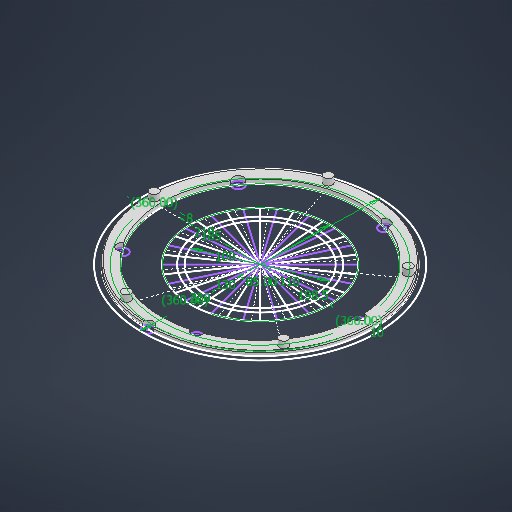
# Autodesk Inventor part: Aparatus_Motion_Conveyer
Saved by Autodesk Inventor 2026.2 (Build 302298000, 298)
## iProperties
Created: 2025-12-30
Part Number: Aparatus_Motion_Conveyer
Material: Generic
Document SubType Name: Modeling
Designer: Cobble
Density: 1 g/cm^3
Appearance: Default
Author: Cobble
Autodesk Inventor part; units mm, degrees
ref_plane "YZ Plane" through (0, 0, 0) normal (1, 0, 0) x (0, 1, 0)
ref_plane "XZ Plane" through (0, 0, 0) normal (0, 1, 0) x (-1, 0, 0)
ref_plane "XY Plane" through (0, 0, 0) normal (0, 0, 1) x (1, 0, 0)
sketch "Sketch1" plane through (0, 0, 0) normal (0, 0, 1) x (1, 0, 0)
  circle A0 centre (0, 0) radius 99.25
  circle A1 centre (-99.25, 0) radius 4
  circle A2 centre (0, 0) radius 92.5
  circle A3 centre (0, 0) radius 105
  line L0 (0, 0) -> (-99.25, 0) construction
  line L1 (0, 0) -> (-30.6699, -94.3924) construction
  circle A4 centre (-30.6699, -94.3924) radius 4
  line L2 (0, 0) -> (80.2949, -58.3377) construction
  circle A5 centre (80.2949, -58.3377) radius 4
  line L3 (0, 0) -> (80.2949, 58.3377) construction
  circle A6 centre (80.2949, 58.3377) radius 4
  line L4 (0, 0) -> (-30.6699, 94.3924) construction
  circle A7 centre (-30.6699, 94.3924) radius 4
  circle A8 centre (0, 0) radius 50
  circle A9 centre (0, 0) radius 55
  circle A10 centre (0, 0) radius 65
  line L5 (0, 0) -> (0, -65) construction
  line L6 (0, 0) -> (5.6651, -64.7527)
  line L7 (0, 0) -> (65, 0) construction
  line L8 (0, 0) -> (-5.6651, -64.7527)
  line L9 (0, 0) -> (16.8232, -62.7852)
  line L10 (0, 0) -> (22.2313, -61.08) construction
  line L11 (0, 0) -> (27.4702, -58.91)
  line L12 (0, 0) -> (37.2825, -53.2449)
  line L13 (0, 0) -> (41.7812, -49.7929) construction
  line L14 (0, 0) -> (45.9619, -45.9619)
  line L15 (0, 0) -> (53.2449, -37.2825)
  line L16 (0, 0) -> (56.2917, -32.5) construction
  line L17 (0, 0) -> (58.91, -27.4702)
  line L18 (0, 0) -> (62.7852, -16.8232)
  line L19 (0, 0) -> (64.0125, -11.2871) construction
  line L20 (0, 0) -> (64.7527, -5.6651)
  line L21 (0, 0) -> (64.7527, 5.6651)
  line L22 (0, 0) -> (64.0125, 11.2871) construction
  line L23 (0, 0) -> (62.7852, 16.8232)
  line L24 (0, 0) -> (58.91, 27.4702)
  line L25 (0, 0) -> (56.2917, 32.5) construction
  line L26 (0, 0) -> (53.2449, 37.2825)
  line L27 (0, 0) -> (45.9619, 45.9619)
  line L28 (0, 0) -> (41.7812, 49.7929) construction
  line L29 (0, 0) -> (37.2825, 53.2449)
  line L30 (0, 0) -> (27.4702, 58.91)
  line L31 (0, 0) -> (22.2313, 61.08) construction
  line L32 (0, 0) -> (16.8232, 62.7852)
  line L33 (0, 0) -> (5.6651, 64.7527)
  line L34 (0, 0) -> (0, 65) construction
  line L35 (0, 0) -> (-5.6651, 64.7527)
  line L36 (0, 0) -> (-16.8232, 62.7852)
  line L37 (0, 0) -> (-22.2313, 61.08) construction
  line L38 (0, 0) -> (-27.4702, 58.91)
  line L39 (0, 0) -> (-37.2825, 53.2449)
  line L40 (0, 0) -> (-41.7812, 49.7929) construction
  line L41 (0, 0) -> (-45.9619, 45.9619)
  line L42 (0, 0) -> (-53.2449, 37.2825)
  line L43 (0, 0) -> (-56.2917, 32.5) construction
  line L44 (0, 0) -> (-58.91, 27.4702)
  line L45 (0, 0) -> (-62.7852, 16.8232)
  line L46 (0, 0) -> (-64.0125, 11.2871) construction
  line L47 (0, 0) -> (-64.7527, 5.6651)
  line L48 (0, 0) -> (-64.7527, -5.6651)
  line L49 (0, 0) -> (-64.0125, -11.2871) construction
  line L50 (0, 0) -> (-62.7852, -16.8232)
  line L51 (0, 0) -> (-58.91, -27.4702)
  line L52 (0, 0) -> (-56.2917, -32.5) construction
  line L53 (0, 0) -> (-53.2449, -37.2825)
  line L54 (0, 0) -> (-45.9619, -45.9619)
  line L55 (0, 0) -> (-41.7812, -49.7929) construction
  line L56 (0, 0) -> (-37.2825, -53.2449)
  line L57 (0, 0) -> (-27.4702, -58.91)
  line L58 (0, 0) -> (-22.2313, -61.08) construction
  line L59 (0, 0) -> (-16.8232, -62.7852)
  circle A11 centre (0, 0) radius 110
  circle A12 centre (0, -105) radius 5
  circle A13 centre (92.5, 0) radius 5
  circle A14 centre (28.5841, 87.9727) radius 5
  circle A15 centre (-74.8341, 54.3701) radius 5
  circle A16 centre (-74.8341, -54.3701) radius 5
  circle A17 centre (28.5841, -87.9727) radius 5
  point P0 (0, -50)
  point P1 (53.1259, -14.235)
  point P2 (49.8469, -23.244)
  point P3 (45.0534, -31.5467)
  point P4 (38.8909, -38.8909)
  point P5 (31.5467, -45.0534)
  point P6 (23.244, -49.8469)
  point P7 (14.235, -53.1259)
  point P8 (4.7936, -54.7907)
  point P9 (-14.235, -53.1259)
  point P10 (-4.7936, -54.7907)
  point P11 (-23.244, -49.8469)
  point P12 (-31.5467, -45.0534)
  point P13 (-38.8909, -38.8909)
  point P14 (-45.0534, -31.5467)
  point P15 (-49.8469, -23.244)
  point P16 (-53.1259, -14.235)
  point P17 (-54.7907, -4.7936)
  point P18 (-54.7907, 4.7936)
  point P19 (-53.1259, 14.235)
  point P20 (-49.8469, 23.244)
  point P21 (-45.0534, 31.5467)
  point P22 (-38.8909, 38.8909)
  point P23 (-31.5467, 45.0534)
  point P24 (-23.244, 49.8469)
  point P25 (-14.235, 53.1259)
  point P26 (-4.7936, 54.7907)
  point P27 (4.7936, 54.7907)
  point P28 (14.235, 53.1259)
  point P29 (23.244, 49.8469)
  point P30 (31.5467, 45.0534)
  point P31 (38.8909, 38.8909)
  point P32 (45.0534, 31.5467)
  point P33 (49.8469, 23.244)
  point P34 (53.1259, 14.235)
  point P35 (54.7907, 4.7936)
  point P36 (54.7907, -4.7936)
  point P37 (-4.9986, -104.881)
  point P38 (4.9986, -104.881)
  point P39 (92.3649, 4.9982)
  point P40 (92.3649, -4.9982)
  point P41 (33.2959, -86.2997)
  point P42 (23.7888, -89.3887)
  point P43 (-71.7869, -58.3343)
  point P44 (-77.6626, -50.2471)
  point P45 (-77.6626, 50.2471)
  point P46 (-71.7869, 58.3343)
  point P47 (23.7888, 89.3887)
  point P48 (33.2959, 86.2997)
  dimension "d0" = 198.5
  dimension "d2" = 185
  dimension "d3" = 210
  dimension "d14" = 100
  dimension "d17" = 110
  dimension "d25" = 130
  dimension "d1" = 8
  dimension "d6" = 360
  dimension "d26" = 85
  dimension "d29" = 360
  dimension "d44" = 220
  dimension "d65" = 10
  dimension "d72" = 360
  constraints: 120 end point, 12 centre point, 9 coincident, 2 horizontal, 1 equal length, 1 horizontal alignment, 1 vertical, 1 vertical alignment, 192 other
  measures "d1" diameter of A1
  measures "d26" angle of L6 L7
  measures "d44" diameter of A11
  measures "d65" diameter of A13
extrude "Extrusion1" add sketch "Sketch1" along normal blind 4 contours A0 A5 A4 A1 A7 A6 | A3 A12 picked at (-81.8104, -62.3728)
extrude "Extrusion2" add sketch "Sketch1" along normal blind 10 contours A6 A0 | A0 A6 | A5 A0 | A0 A5 | A7 A0 | A0 A7 | A4 A0 | A0 A4 | A1 A0 | A0 A1
chamfer "Chamfer6" distance 1 angle 45 1 edges at (0, 105, 4)
body "Solid1"
